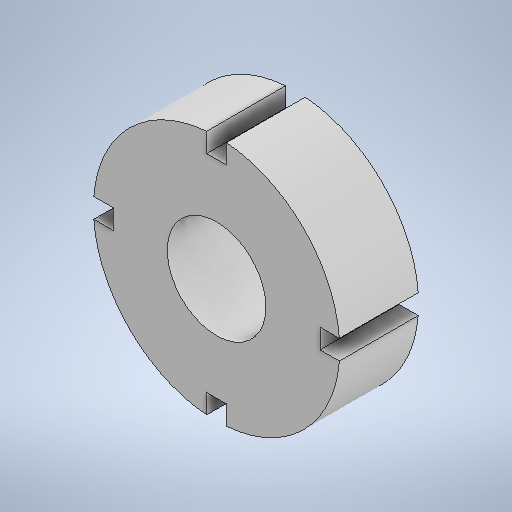
# Autodesk Inventor part: Cubierta de acoplamiento
Saved by Autodesk Inventor 2025.3 (Build 293356030, 356C)
## iProperties
Created: 2025-08-24
Part Number: Cubierta de acoplamiento
Material: Generic
Document SubType Name: Modeling
Designer: PC
Density: 1 g/cm^3
Appearance: Default
Author: PC
Autodesk Inventor part; units mm, degrees
ref_plane "YZ Plane" through (0, 0, 0) normal (1, 0, 0) x (0, 1, 0)
ref_plane "XZ Plane" through (0, 0, 0) normal (0, 1, 0) x (-1, 0, 0)
ref_plane "XY Plane" through (0, 0, 0) normal (0, 0, 1) x (1, 0, 0)
sketch "Sketch1" plane through (0, 0, 0) normal (0, 0, 1) x (1, 0, 0)
  circle A0 centre (0, 0) radius 5
  line L0 (-12.4599, 1) -> (-10.5, 1)
  line L1 (-10.5, 1) -> (-10.5, -1)
  line L2 (-10.5, -1) -> (-12.4599, -1)
  line L3 (-14.5, 1) -> (-10.5, -1) construction
  line L4 (-10.5, 1) -> (-14.5, -1) construction
  line L5 (1, 12.4599) -> (1, 10.5)
  line L6 (1, 10.5) -> (-1, 10.5)
  line L7 (-1, 10.5) -> (-1, 12.4599)
  line L8 (-1, 14.5) -> (1, 10.5) construction
  line L9 (1, 14.5) -> (-1, 10.5) construction
  line L10 (10.5, 1) -> (12.4599, 1)
  line L11 (12.4599, -1) -> (10.5, -1)
  line L12 (10.5, -1) -> (10.5, 1)
  line L13 (10.5, 1) -> (14.5, -1) construction
  line L14 (14.5, 1) -> (10.5, -1) construction
  line L15 (1, -12.4599) -> (1, -10.5)
  line L16 (1, -10.5) -> (-1, -10.5)
  line L17 (-1, -10.5) -> (-1, -12.4599)
  line L18 (-1, -14.5) -> (1, -10.5) construction
  line L19 (1, -14.5) -> (-1, -10.5) construction
  arc A1 (-1, 12.4599) -> (-12.4599, 1) centre (0, 0) ccw
  arc A2 (12.4599, 1) -> (1, 12.4599) centre (0, 0) ccw
  arc A3 (-12.4599, -1) -> (-1, -12.4599) centre (0, 0) ccw
  arc A4 (1, -12.4599) -> (12.4599, -1) centre (0, 0) ccw
  dimension "d0" = 10
  dimension "d10" = 21
  constraints: 40 end point, 8 point on circle, 5 centre point, 4 parallel, 2 coincident, 2 horizontal, 1 perpendicular
  measures "d0" diameter of A0
  measures "d10" distance of L10.start L0.end
extrude "Extrusion1" add sketch "Sketch1" along normal blind 8
body "Solid1"
